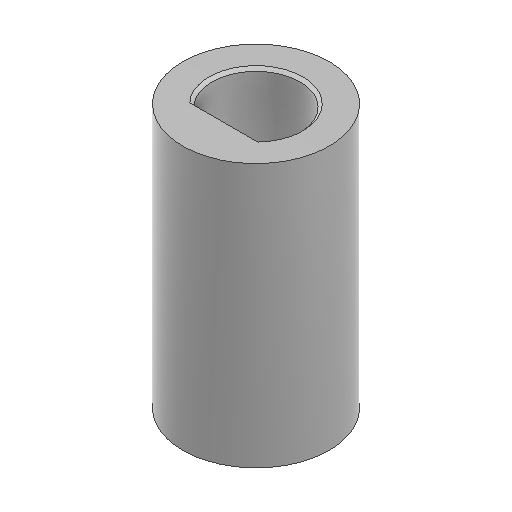
# Autodesk Inventor part: Шкив для ДПТ
Saved by Autodesk Inventor 2022 (Build 260153000, 153)
## iProperties
Created: 2023-02-20
Part Number: Шкив для ДПТ
Material: Типовые
Document SubType Name: Modeling
Designer: Глеб
Density: 1 g/cm^3
Appearance: По умолчанию
Author: Глеб
Autodesk Inventor part; units mm, degrees
ref_plane "YZ Plane" through (0, 0, 0) normal (1, 0, 0) x (0, 1, 0)
ref_plane "XZ Plane" through (0, 0, 0) normal (0, 1, 0) x (-1, 0, 0)
ref_plane "XY Plane" through (0, 0, 0) normal (0, 0, 1) x (1, 0, 0)
sketch "Эскиз1" plane through (0, 0, 0) normal (0, 1, 0) x (-1, 0, 0)
  circle A0 centre (0, 0) radius 1.5
  line L0 (-1.118, 1) -> (1.118, 1)
  circle A1 centre (0, 0) radius 2.5
  dimension "d0" = 3
  dimension "d11" = 2.236
  dimension "d12" = 5
  constraints: 2 centre point, 2 coincident, 2 end point, 2 point on circle, 1 horizontal
  measures "d0" diameter of A0
  measures "d11" distance of L0.start L0.end
  measures "d12" diameter of A1
extrude "Выдавливание4" add sketch "Эскиз1" along normal blind 9 contours L0 A0 | A1 picked at (-0.0599, 1.1631)
chamfer "Фаска1" distance 0.1 angle 45 4 edges at (0, 0, -1.5) (0, 0, 1) (0, 9, 1) (0, 9, -1.5)
